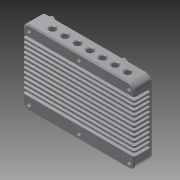
# Autodesk Inventor part: nanopi_m4_heatsink
Saved by Autodesk Inventor 2013 SP2 (Build 170200200, 200)
## iProperties
Created: 2018-09-18
Part Number: nanopi_m4_heatsink
Material: Generic
Document SubType Name: Modeling
Designer: alex
Density: 1 g/cm^3
Mass: 50.1474 g
Surface Area: 444.443 cm^2
Volume: 50.1474 cm^3
Author: alex
Autodesk Inventor part; units mm, degrees
ref_plane "YZ Plane" through (0, 0, 0) normal (1, 0, 0) x (0, 1, 0)
ref_plane "XZ Plane" through (0, 0, 0) normal (0, 1, 0) x (-1, 0, 0)
sketch "Sketch1" plane through (0, 0, 0) normal (0, 1, 0) x (-1, 0, 0)
  line L0 (0, 0) -> (85, 0)
  line L1 (85, 0) -> (85, 56)
  line L2 (85, 56) -> (0, 56)
  line L3 (0, 56) -> (0, 0)
  dimension "d0" = 85
  dimension "d2" = 56
  constraints: 8 end point, 2 parallel, 1 horizontal, 1 perpendicular
  measures "d0" distance of L1.end L2.end
  measures "d2" distance of L2.end L0.start
extrude "Extrusion1" add sketch "Sketch1" along normal blind 1.5
fillet "Fillet1" radius 3 4 edges at (0, 0.75, 56) (0, 0.75, 0) (-85, 0.75, 0) (-85, 0.75, 56)
sketch "Sketch2" plane through (0, 0, 0) normal (0, -1, 0) x (1, 0, 0)
  arc A0 (-82, 56) -> (-85, 53) centre (-82, 53) ccw projected
  line L0 (-85, 3) -> (-85, 53) projected
  arc A1 (-85, 3) -> (-82, 0) centre (-82, 3) ccw projected
  line L1 (-3, 0) -> (-82, 0) projected
  arc A2 (-3, 0) -> (0, 3) centre (-3, 3) ccw projected
  line L2 (0, 53) -> (0, 3) projected
  arc A3 (0, 53) -> (-3, 56) centre (-3, 53) ccw projected
  line L3 (-82, 56) -> (-3, 56) projected
  arc A4 (2, 53) -> (-3, 58) centre (-3, 53) ccw
  line L4 (2, 53) -> (2, 3)
  arc A5 (-3, -2) -> (2, 3) centre (-3, 3) ccw
  line L5 (-3, -2) -> (-82, -2)
  arc A6 (-87, 3) -> (-82, -2) centre (-82, 3) ccw
  line L6 (-87, 3) -> (-87, 53)
  arc A7 (-82, 58) -> (-87, 53) centre (-82, 53) ccw
  line L7 (-82, 58) -> (-3, 58)
  point P0 (0, 0)
  dimension "d6" = 2
  constraints: 8 end point, 8 point on circle, 4 centre point, 7 other
  measures "d6" distance between parallel lines of L3 L7
extrude "Extrusion2" add sketch "Sketch2" along normal blind 14 contours L3 A3 L2 A2 L1 A1 L0 A0 | L4 A5 L5 A6 L6 A7 L7 A4
sketch "Sketch3" plane through (0, 1.5, 0) normal (0, 1, 0) x (1, 0, 0)
  line L0 (-82, -56) -> (-3, -56) projected
  line L1 (-3, 0) -> (-82, 0) projected
  line L2 (-85, -3) -> (-85, -53) projected
  circle A0 centre (-81.5, -3.5) radius 2.5
  circle A1 centre (-23.5, -3.5) radius 2.5
  circle A2 centre (-81.5, -52.5) radius 2.5
  circle A3 centre (-23.5, -52.5) radius 2.5
  point P0 (0, 0)
  dimension "d9" = 5
  dimension "d10" = 3.5
  dimension "d11" = 3.5
  dimension "d12" = 5
  dimension "d13" = 3.5
  dimension "d14" = 58
  dimension "d15" = 5
  dimension "d16" = 3.5
  dimension "d17" = 3.5
  dimension "d18" = 5
  dimension "d19" = 58
  dimension "d20" = 3.5
  dimension "d77" = 49
  constraints: 4 centre point
  measures "d9" diameter of A0
  measures "d10" distance from line of L1 A0.centre
  measures "d11" distance from line of L2 A0.centre
  measures "d12" diameter of A1
  measures "d13" distance from line of L1 A1.centre
  measures "d14" distance of A0.centre A1.centre
  measures "d15" diameter of A2
  measures "d16" distance from line of L2 A2.centre
  measures "d17" distance from line of A2.centre L0
  measures "d18" diameter of A3
  measures "d19" distance of A2.centre A3.centre
  measures "d20" distance from line of L0 A3.centre
  measures "d77" distance of A0.centre A2.centre
extrude "Extrusion3" add sketch "Sketch3" along normal blind 3
sketch "Sketch4" plane through (-81.5, 4.5, 52.5) normal (0, 1, 0) x (1, 0, 0)
  circle A0 centre (0, 0) radius 2.5 projected
  circle A1 centre (0, 49) radius 2.5 projected
  circle A2 centre (58, 49) radius 2.5 projected
  circle A3 centre (58, 0) radius 2.5 projected
  point P0 (81.5, 52.5)
  constraints: 4 coincident
hole "Hole1" at (-81.5, 4.5, 3.5) at (-23.5, 4.5, 3.5) at (-23.5, 4.5, 52.5) at (-81.5, 4.5, 52.5) direction (0, -1, 0) diameter 3 depth 7
chamfer "Chamfer1" distance 1 angle 45 8 edges at (-42.5, -14, -2) (0.5355, -14, -0.5355) (2, -14, 28) (0.5355, -14, 56.5355) (-42.5, -14, 58) (-85.5355, -14, 56.5355) (-87, -14, 28) (-85.5355, -14, -0.5355)
sketch "Sketch5" plane through (0, -14, 0) normal (0, -1, 0) x (1, 0, 0)
  line L0 (-3, -1) -> (-82, -1) projected
  line L1 (-82, 57) -> (-3, 57) projected
  line L2 (1, 53) -> (1, 3) projected
  line L3 (-86, 3) -> (-86, 53) projected
  line L4 (-42.5, 53.5) -> (-42.5, 57)
  line L5 (-42.5, 2.5) -> (-42.5, -1)
  line L6 (-82.5, 53.5) -> (-86, 53.5)
  line L7 (-2.5, 53.5) -> (1, 53.5)
  point P0 (0, 0)
  point P1 (-82.5, 2.5)
  point P2 (-2.5, 2.5)
  dimension "d80" = 40
  dimension "d83" = 51
  constraints: 8 end point, 3 collinear, 3 perpendicular, 2 midpoint, 2 point on line, 1 horizontal, 1 vertical, 5 other
  measures "d80" distance of L6.start L4.start
  measures "d83" distance of L6.start point (-82.5, 2.5)
hole "Hole2" at (-82.5, -14, 53.5) at (-42.5, -14, 53.5) at (-2.5, -14, 53.5) at (-2.5, -14, 2.5) at (-42.5, -14, 2.5) at (-82.5, -14, 2.5) direction (0, 1, 0) diameter 3 depth 4.5 countersink diameter 3.5 countersink angle 90
sketch "Sketch6" plane through (-3, 0, -2) normal (0, 0, -1) x (-1, 0, 0)
  line L0 (0, 0) -> (79, 0) projected
  line L1 (79, 0) -> (79, -13) projected
  line L2 (-5, 0) -> (-5, -13) projected
  line L3 (84, 0) -> (84, -13) projected
  line L4 (7, -7) -> (-5, -7)
  line L5 (67, -7) -> (79, -7)
  point P0 (-3, 0)
  point P1 (57, -7)
  point P2 (47, -7)
  point P3 (37, -7)
  point P4 (27, -7)
  point P5 (17, -7)
  dimension "d42" = 10
  constraints: 4 end point, 2 perpendicular, 2 point on line, 1 collinear, 1 horizontal, 6 other
  measures "d42" distance of L5.start point (57, -7)
hole "Hole3" at (-70, -7, -2) at (-60, -7, -2) at (-50, -7, -2) at (-40, -7, -2) at (-30, -7, -2) at (-20, -7, -2) at (-10, -7, -2) direction (0, 0, 1) diameter 5 depth 8 countersink diameter 6.2 countersink angle 90
ref_plane "Work Plane1" through (-3, 0, 28) normal (0, 0, -1) x (-1, 0, 0)
mirror "Mirror1" about plane through (-3, 0, 28) normal (0, 0, -1) of "Hole3"
sketch "Sketch7" plane through (0, -14, 0) normal (0, -1, 0) x (1, 0, 0)
  line L0 (-3, -1) -> (-82, -1) projected
  line L1 (-82, 57) -> (-3, 57) projected
  line L2 (-86, 3) -> (-86, 53) projected
  line L3 (-99.6358, 45.6667) -> (9.9097, 45.6667)
  line L4 (9.9097, 45.6667) -> (9.9097, 43.6667)
  line L5 (9.9097, 43.6667) -> (-99.6358, 43.6667)
  line L6 (-99.6358, 43.6667) -> (-99.6358, 45.6667)
  line L7 (-99.6358, 42.1667) -> (9.9097, 42.1667)
  line L8 (9.9097, 42.1667) -> (9.9097, 40.1667)
  line L9 (9.9097, 40.1667) -> (-99.6358, 40.1667)
  line L10 (-99.6358, 40.1667) -> (-99.6358, 42.1667)
  line L11 (-99.6358, 38.6667) -> (9.9097, 38.6667)
  line L12 (9.9097, 38.6667) -> (9.9097, 36.6667)
  line L13 (9.9097, 36.6667) -> (-99.6358, 36.6667)
  line L14 (-99.6358, 36.6667) -> (-99.6358, 38.6667)
  line L15 (-99.6358, 35.1667) -> (9.9097, 35.1667)
  line L16 (9.9097, 35.1667) -> (9.9097, 33.1667)
  line L17 (9.9097, 33.1667) -> (-99.6358, 33.1667)
  line L18 (-99.6358, 33.1667) -> (-99.6358, 35.1667)
  line L19 (-99.6358, 31.6667) -> (9.9097, 31.6667)
  line L20 (9.9097, 31.6667) -> (9.9097, 29.6667)
  line L21 (9.9097, 29.6667) -> (-99.6358, 29.6667)
  line L22 (-99.6358, 29.6667) -> (-99.6358, 31.6667)
  line L23 (-99.6358, 28.1667) -> (9.9097, 28.1667)
  line L24 (9.9097, 28.1667) -> (9.9097, 26.1667)
  line L25 (9.9097, 26.1667) -> (-99.6358, 26.1667)
  line L26 (-99.6358, 26.1667) -> (-99.6358, 28.1667)
  line L27 (-99.6358, 24.6667) -> (9.9097, 24.6667)
  line L28 (9.9097, 24.6667) -> (9.9097, 22.6667)
  line L29 (9.9097, 22.6667) -> (-99.6358, 22.6667)
  line L30 (-99.6358, 22.6667) -> (-99.6358, 24.6667)
  line L31 (-99.6358, 21.1667) -> (9.9097, 21.1667)
  line L32 (9.9097, 21.1667) -> (9.9097, 19.1667)
  line L33 (9.9097, 19.1667) -> (-99.6358, 19.1667)
  line L34 (-99.6358, 19.1667) -> (-99.6358, 21.1667)
  line L35 (-99.6358, 17.6667) -> (9.9097, 17.6667)
  line L36 (9.9097, 17.6667) -> (9.9097, 15.6667)
  line L37 (9.9097, 15.6667) -> (-99.6358, 15.6667)
  line L38 (-99.6358, 15.6667) -> (-99.6358, 17.6667)
  line L39 (-99.6358, 14.1667) -> (9.9097, 14.1667)
  line L40 (9.9097, 14.1667) -> (9.9097, 12.1667)
  line L41 (9.9097, 12.1667) -> (-99.6358, 12.1667)
  line L42 (-99.6358, 12.1667) -> (-99.6358, 14.1667)
  line L43 (-63.4683, 45.6667) -> (-63.4683, 57)
  line L44 (-63.4683, -1) -> (-63.4683, 10.3333)
  line L45 (-99.6358, 46.9667) -> (9.9097, 46.9667)
  line L46 (9.9097, 46.9667) -> (9.9097, 49.4667)
  line L47 (9.9097, 49.4667) -> (-99.6358, 49.4667)
  line L48 (-99.6358, 49.4667) -> (-99.6358, 46.9667)
  line L49 (-3, 58) -> (-82, 58) projected
  line L50 (-99.6358, 10.8667) -> (9.9097, 10.8667)
  line L51 (9.9097, 10.8667) -> (9.9097, 8.3667)
  line L52 (9.9097, 8.3667) -> (-99.6358, 8.3667)
  line L53 (-99.6358, 8.3667) -> (-99.6358, 10.8667)
  point P0 (0, 0)
  dimension "d55" = 2
  dimension "d60" = 3.5
  dimension "d72" = 2.5
  dimension "d74" = 1.3
  dimension "d75" = 1.3
  dimension "d76" = 2.5
  constraints: 100 end point, 6 parallel, 4 perpendicular, 3 horizontal, 3 point on line, 1 collinear, 1 vertical, 72 other
  measures "d55" distance of L5.end L3.start
  measures "d60" distance of L3.end L8.start
  measures "d72" distance of L47.end L45.start
  measures "d74" distance between parallel lines of L3 L45
  measures "d75" distance between parallel lines of L50 L41
  measures "d76" distance of L52.end L50.start
extrude "Extrusion4" cut sketch "Sketch7" against normal blind 13 contours L52 L53 L50 L2 | L2 L50 L51 L52 | L5 L6 L3 L2 | L2 L3 L4 L5 | L9 L10 L7 L2 | L2 L7 L8 L9 | L13 L14 L11 L2 | L2 L11 L12 L13 | L17 L18 L15 L2 | L2 L15 L16 L17 | L21 L22 L19 L2 | L2 L19 L20 L21 | L25 L26 L23 L2 | L2 L23 L24 L25 | L29 L30 L27 L2 | L2 L27 L28 L29 | L33 L34 L31 L2 | L2 L31 L32 L33 | L37 L38 L35 L2 | L2 L35 L36 L37 | L41 L42 L39 L2 | L2 L39 L40 L41 | L45 L48 L47 L2 | L2 L47 L43 L45 | L43 L47 L46 L45
body "Solid1"
